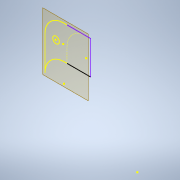
# Autodesk Inventor part: adapter2
Saved by Autodesk Inventor 2020.1 (Build 241239000, 239)
## iProperties
Created: 2019-10-25
Part Number: adapter2
Material: Generic
Document SubType Name: Modeling
Designer: jesse
Density: 1 g/cm^3
Appearance: Default
Author: jesse
Autodesk Inventor part; units mm, degrees
ref_plane "YZ Plane" through (0, 0, 0) normal (1, 0, 0) x (0, 1, 0)
ref_plane "XZ Plane" through (0, 0, 0) normal (0, 1, 0) x (-1, 0, 0)
ref_plane "XY Plane" through (0, 0, 0) normal (0, 0, 1) x (1, 0, 0)
ref_plane "Work Plane2" through (0, 0, 0) normal (0, 0, 1) x (1, 0, 0)
sketch "Sketch3" plane through (0, 0, 0) normal (0, 0, 1) x (1, 0, 0)
  line L0 (-24.13, 20.32) -> (-25.146, 20.32) projected
  arc A0 (-25.146, 20.32) -> (-31.75, 13.716) centre (-25.146, 13.716) ccw projected
  line L1 (-31.75, 13.716) -> (-31.75, 6.096) projected
  arc A1 (-25.146, 12.7) -> (-31.75, 6.096) centre (-25.146, 6.096) ccw projected
  line L2 (-24.13, 12.7) -> (-25.146, 12.7) projected
  line L3 (-24.13, 20.32) -> (-24.13, 12.7) construction
  circle A2 centre (-27.94, 15.24) radius 1.1303 projected
  line L4 (-24.13, 12.7) -> (-17.13, 12.7)
  line L5 (-17.13, 12.7) -> (-17.13, 20.32)
  line L6 (-17.13, 20.32) -> (-24.13, 20.32)
  line L7 (-24.13, 20.32) -> (-24.13, 20.2414)
  line L8 (-24.13, 12.7) -> (-31.75, 12.7)
  point P0 (0, 0)
  dimension "d0" = 7
  constraints: 10 end point, 2 horizontal, 2 parallel, 1 collinear, 1 perpendicular, 1 point on circle, 1 point on line
  measures "d0" distance from line of L0.start L5
extrude "Extrusion1" add sketch "Sketch3" along normal blind 3.175 contours L6 L5 L4 L2 L8 L1 A0 L0
sketch "Sketch4" plane through (0, 0, 0) normal (0, 0, -1) x (-1, 0, 0)
  line L0 (20.13, 20.32) -> (20.13, 12.7) construction
  line L1 (22.13, 12.7) -> (22.13, 20.32) construction
  line L2 (17.13, 20.32) -> (25.146, 20.32) projected
  line L3 (31.75, 12.7) -> (17.13, 12.7) projected
  line L4 (20.03, 20.32) -> (18.23, 20.32)
  line L5 (18.23, 20.32) -> (18.23, 12.7)
  line L6 (18.23, 12.7) -> (20.03, 12.7)
  line L7 (20.03, 12.7) -> (20.03, 20.32)
  line L8 (22.23, 20.32) -> (24.03, 20.32)
  line L9 (24.03, 20.32) -> (24.03, 12.7)
  line L10 (24.03, 12.7) -> (22.23, 12.7)
  line L11 (22.23, 12.7) -> (22.23, 20.32)
  line L12 (24.13, 20.32) -> (24.13, 12.7) construction
  point P0 (0, 0)
  dimension "d3" = 0.1
  dimension "d4" = 0.1
  dimension "d6" = 0.1
  constraints: 16 end point, 4 parallel, 4 point on line, 2 horizontal, 2 perpendicular, 1 collinear
  measures "d3" distance between parallel lines of L7 L0
  measures "d4" distance between parallel lines of L11 L1
  measures "d6" distance between parallel lines of L12 L9
extrude "Extrusion2" add sketch "Sketch4" along normal blind 6.35 contours L2 L7 L3 L5 | L2 L9 L3 L11
sketch "Sketch5" plane through (-18.23, 12.7, 0) normal (1, 0, 0) x (0, 0, -1)
  line L0 (0, 1.016) -> (0, 0) projected
  line L1 (6.35, 0) -> (6.35, 7.62) projected
  line L2 (0, 0) -> (6.35, 7.62) construction
  circle A0 centre (3.175, 3.81) radius 1.5875
  point P0 (0, -12.7)
  dimension "d9" = 3.175
  constraints: 2 end point, 1 centre point, 1 midpoint
  measures "d9" diameter of A0
extrude "Extrusion3" cut sketch "Sketch5" against normal blind 9.75
body "Solid1"
